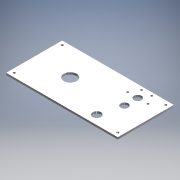
# Autodesk Inventor part: V2 Plate 1
Saved by Autodesk Inventor 2019.4 (Build 234330000, 330)
## iProperties
Created: 2020-03-11
Part Number: V2 Plate 1
Material: Aluminum 6061
Document SubType Name: Modeling
Designer: Mark
Mass: 526.027 g
Surface Area: 824.655 cm^2
Volume: 194.825 cm^3
Density: 2.7 g/cm^3
Appearance: Aluminum - Flat
Author: Mark
Autodesk Inventor part; units mm, degrees
ref_plane "YZ Plane" through (0, 0, 0) normal (1, 0, 0) x (0, 1, 0)
ref_plane "XZ Plane" through (0, 0, 0) normal (0, 1, 0) x (-1, 0, 0)
ref_plane "XY Plane" through (0, 0, 0) normal (0, 0, 1) x (1, 0, 0)
sketch "Sketch1" plane through (0, 0, 0) normal (0, 1, 0) x (-1, 0, 0)
  line L0 (0, 0) -> (279, 0)
  line L1 (279, 0) -> (279, -140)
  line L2 (279, -140) -> (0, -140)
  line L3 (0, -140) -> (0, 0)
  circle A0 centre (10, -10) radius 2.75
  circle A1 centre (10, -130) radius 2.75
  circle A2 centre (269, -10) radius 2.75
  circle A3 centre (269, -130) radius 2.75
  dimension "d0" = 279
  dimension "d1" = 140
  dimension "d2" = 5.5
  dimension "d3" = 5.5
  dimension "d4" = 5.5
  dimension "d5" = 5.5
  dimension "d6" = 10
  dimension "d7" = 10
  dimension "d8" = 10
  dimension "d9" = 10
  dimension "d10" = 10
  dimension "d11" = 10
  dimension "d12" = 10
  dimension "d13" = 10
  constraints: 8 end point, 4 centre point, 2 parallel, 1 horizontal, 1 perpendicular
  measures "d0" distance of L1.end L2.end
  measures "d1" distance of L0.end L1.end
  measures "d2" diameter of A0
  measures "d3" diameter of A1
  measures "d4" diameter of A2
  measures "d5" diameter of A3
  measures "d6" distance from line of L2 A3.centre
  measures "d7" distance from line of L1 A3.centre
  measures "d8" distance from line of L1 A2.centre
  measures "d9" distance from line of L0 A2.centre
  measures "d10" distance from line of L3 A0.centre
  measures "d11" distance from line of A0.centre L0
  measures "d12" distance from line of L3 A1.centre
  measures "d13" distance from line of L2 A1.centre
extrude "Extrusion1" add sketch "Sketch1" along normal blind 5
sketch "Sketch2" plane through (0, 0, 0) normal (0, -1, 0) x (1, 0, 0)
  circle A0 centre (-60, -110) radius 9.575
  line L0 (-279, -140) -> (0, -140) projected
  line L1 (0, -140) -> (0, 0) projected
  line L2 (-60, -110) -> (-60, -76.98) construction
  circle A1 centre (-60, -76.98) radius 9.5
  circle A2 centre (-60, -110) radius 25.4 construction
  circle A3 centre (-34.6, -110) radius 2.6
  circle A4 centre (-60, -110) radius 25.4 construction
  circle A5 centre (-47.3, -88.003) radius 2.6
  circle A6 centre (-60, -110) radius 25.4 construction
  circle A7 centre (-72.7, -88.003) radius 2.6
  circle A8 centre (-60, -110) radius 25.4 construction
  circle A9 centre (-85.4, -110) radius 2.6
  circle A10 centre (-60, -110) radius 25.4 construction
  circle A11 centre (-72.7, -131.997) radius 2.6
  circle A12 centre (-60, -110) radius 25.4 construction
  circle A13 centre (-47.3, -131.997) radius 2.6
  line L3 (-60, -110) -> (-59, -110) construction
  line L4 (-60, -110) -> (-30, -110) construction
  line L5 (-60, -110) -> (-30, -110) construction
  circle A14 centre (-75, -22.7669) radius 10.5
  line L6 (-60, -76.98) -> (-75, -22.7669) construction
  line L7 (-75, -22.7669) -> (-188.9701, -70) construction
  line L8 (-279.0043, -70) -> (0, -70) construction
  line L9 (0, 0) -> (0, -140) projected
  circle A15 centre (-188.9701, -70) radius 16
  dimension "d23" = 50.8
  dimension "d16" = 19.15
  dimension "d17" = 30
  dimension "d18" = 60
  dimension "d19" = 33.02
  dimension "d20" = 19
  dimension "d24" = 5.2
  dimension "d27" = 360
  dimension "d31" = 30
  dimension "d32" = 0
  dimension "d33" = 21
  dimension "d34" = 56.25
  dimension "d35" = 15
  dimension "d36" = 123.37
  dimension "d37" = 32
  constraints: 14 end point, 10 centre point, 4 coincident, 2 horizontal, 2 horizontal alignment, 2 parallel, 2 point on line, 1 collinear, 1 midpoint, 41 other
  measures "d16" diameter of A0
  measures "d17" distance from line of L0 L2.start
  measures "d18" distance from line of L1 L2.start
  measures "d19" distance of L2.start L2.end
  measures "d20" diameter of A1
  measures "d24" diameter of A3
  measures "d31" distance of L3.start L4.end
  measures "d32" distance between parallel lines of L4 L5
  measures "d33" diameter of A14
  measures "d34" distance of L6.start L6.end
  measures "d35" horizontal distance of L6.start A14.centre
  measures "d36" distance of L6.end L7.end
  measures "d37" diameter of A15
extrude "Extrusion2" cut sketch "Sketch2" against normal blind 5 contours A0 | A1 | A3 | A9 | A11 | A13 | A14 | A15
body "Solid1"
